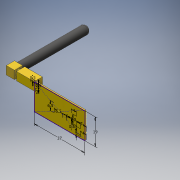
# Autodesk Inventor part: APC 220
Saved by Autodesk Inventor 2016 (Build 200138000, 138)
## iProperties
Created: 2016-05-08
Part Number: APC 220
Material: Generic
Document SubType Name: Modeling
Designer: Kenneth Daniel
Density: 1 g/cm^3
Appearance: Default
Author: Kenneth Daniel
Autodesk Inventor part; units mm, degrees
ref_plane "YZ Plane" through (0, 0, 0) normal (1, 0, 0) x (0, 1, 0)
ref_plane "XZ Plane" through (0, 0, 0) normal (0, 1, 0) x (-1, 0, 0)
ref_plane "XY Plane" through (0, 0, 0) normal (0, 0, 1) x (1, 0, 0)
sketch "Sketch1" plane through (0, 0, 0) normal (0, 1, 0) x (-1, 0, 0)
  line L0 (-18.5, 9.5) -> (-18.5, -9.5)
  line L1 (-18.5, -9.5) -> (18.5, -9.5)
  line L2 (18.5, -9.5) -> (18.5, 9.5)
  line L3 (18.5, 9.5) -> (-18.5, 9.5)
  line L4 (-18.5, 9.5) -> (18.5, -9.5) construction
  line L5 (-18.5, -9.5) -> (18.5, 9.5) construction
  point P0 (0, 0)
  dimension "d0" = 19
  dimension "d1" = 37
  constraints: 12 end point, 2 midpoint, 2 parallel, 1 perpendicular, 1 vertical
  measures "d0" distance of L0.start L0.end
  measures "d1" distance of L1.end L0.end
extrude "Extrusion1" add sketch "Sketch1" along normal blind 1
sketch "Sketch2" plane through (0, 1, 0) normal (0, 1, 0) x (1, 0, 0)
  line L0 (-18.5, 9.5) -> (-18.5, -9.5) construction
  line L1 (18.5, 9.5) -> (-18.5, 9.5) construction
  line L2 (-18.5, -9.5) -> (18.5, 9.5) construction
  line L3 (18.5, -9.5) -> (18.5, 9.5) construction
  line L4 (-18.5, 9.5) -> (18.5, -9.5) construction
  line L5 (-18.5, 0) -> (18.5, 0) construction
  line L6 (0, -9.5) -> (0, 9.5) construction
  line L7 (18.5, 9.5) -> (14.5, 9.5) construction
  line L8 (14.5, 9.5) -> (14.5, 8.5) construction
  line L9 (14.5, 8.5) -> (14.5, 4.5)
  line L10 (14.5, 4.5) -> (4.5, 4.5)
  line L11 (4.5, 4.5) -> (4.5, 8.5)
  line L12 (4.5, 8.5) -> (14.5, 8.5)
  line L13 (4.5, 4.5) -> (14.5, 8.5) construction
  line L14 (4.5, 8.5) -> (14.5, 4.5) construction
  line L15 (6.6893, 4.5) -> (6.6893, 8.5) construction
  line L16 (6.6893, 5.3757) -> (14.5, 5.3757) construction
  line L17 (12.159, 4.5) -> (12.159, 8.5) construction
  line L18 (6.6893, 6.5) -> (12.159, 6.5) construction
  line L19 (6.6893, 8.5) -> (12.159, 8.5)
  line L20 (12.159, 4.5) -> (6.6893, 4.5)
  arc A0 (6.6893, 8.5) -> (6.6893, 4.5) centre (6.6893, 6.5) ccw
  arc A1 (12.159, 4.5) -> (12.159, 8.5) centre (12.159, 6.5) ccw
  line L21 (18.5, 4.5) -> (11.5, 4.5) construction
  line L22 (11.5, 4.5) -> (11.5, 4) construction
  line L23 (11.5, 4) -> (11.5, -2)
  line L24 (11.5, -2) -> (7.5, -2)
  line L25 (7.5, -2) -> (7.5, 4)
  line L26 (7.5, 4) -> (11.5, 4)
  line L27 (7.5, 4) -> (1.5, 4) construction
  line L28 (1.5, 4) -> (-5, 4)
  line L29 (-5, 4) -> (-5, -2.5)
  line L30 (-5, -2.5) -> (1.5, -2.5)
  line L31 (1.5, -2.5) -> (1.5, 4)
  line L32 (-18.5, -9.5) -> (-18.5, -9)
  line L33 (-18.5, -9) -> (-18.5, -8)
  line L34 (-18.5, -8) -> (-18.5, -7.5)
  line L35 (-18.5, -7.5) -> (-18.5, -6.5)
  line L36 (-18.5, -6.5) -> (-18.5, -6)
  line L37 (-18.5, -6) -> (-18.5, -5)
  line L38 (-18.5, -5) -> (-16.5, -5)
  line L39 (-16.5, -5) -> (-16.5, -9)
  line L40 (-16.5, -9) -> (-18.5, -9)
  line L41 (-18.5, -8) -> (-16.5, -8)
  line L42 (-18.5, -7.5) -> (-16.5, -7.5)
  line L43 (-18.5, -6.5) -> (-16.5, -6.5)
  line L44 (-18.5, -6) -> (-16.5, -6)
  point P0 (0, 0)
  point P1 (9.4242, 6.5)
  dimension "d4" = 4
  dimension "d5" = 1
  dimension "d6" = 4
  dimension "d7" = 10
  dimension "d8" = 7
  dimension "d9" = 0.5
  dimension "d10" = 6
  dimension "d11" = 4
  dimension "d12" = 6
  dimension "d13" = 6.5
  dimension "d14" = 6.5
  dimension "d15" = 0.5
  dimension "d16" = 1
  dimension "d17" = 0.5
  dimension "d18" = 1
  dimension "d19" = 0.5
  dimension "d20" = 1
  dimension "d21" = 2
  constraints: 86 end point, 15 perpendicular, 14 point on line, 9 parallel, 5 midpoint, 4 point on circle, 4 tangent, 2 centre point, 2 vertical, 8 other
  measures "d4" distance of L1.start L7.end
  measures "d5" distance of L7.end L8.end
  measures "d6" distance of L8.end L9.end
  measures "d7" distance of L9.end L10.end
  measures "d8" distance of L21.start L21.end
  measures "d9" distance of L21.end L22.end
  measures "d10" distance of L22.end L23.end
  measures "d11" distance of L23.end L24.end
  measures "d12" distance of L25.end L27.end
  measures "d13" distance of L27.end L28.end
  measures "d14" distance of L29.end L28.end
  measures "d15" distance of L2.start L32.end
  measures "d16" distance of L32.end L33.end
  measures "d17" distance of L33.end L34.end
  measures "d18" distance of L34.end L35.end
  measures "d19" distance of L35.end L36.end
  measures "d20" distance of L36.end L37.end
  measures "d21" distance of L37.end L38.end
extrude "Extrusion2" add sketch "Sketch2" along normal blind 0.25 contours L9 L10 A1 L12 | A1 L10 A0 L12 | A0 L10 L11 L12 | L23 L24 L25 L26 | L31 L30 L29 L28
extrude "Extrusion3" add sketch "Sketch2" along normal blind 1 contours L33 L41 L39 L40 | L35 L43 L39 L42 | L37 L38 L39 L44
sketch "Sketch3" plane through (-18.5, 0, -9.5) normal (-1, 0, 0) x (0, 0, 1)
  line L0 (19, 0) -> (19, 1) projected
  line L1 (19, 0) -> (19, 6)
  line L2 (19, 6) -> (13, 6)
  line L3 (13, 6) -> (13, 0)
  line L4 (0, 0) -> (19, 0) projected
  point P0 (9.5, 0)
  dimension "d26" = 6
  dimension "d27" = 6
  constraints: 6 end point, 2 perpendicular, 1 collinear, 1 point on line
  measures "d26" distance of L0.start L1.end
  measures "d27" distance of L1.end L2.end
extrude "Extrusion4" add sketch "Sketch3" along normal blind 13
sketch "Sketch4" plane through (-31.5, 0, -9.5) normal (-1, 0, 0) x (0, 0, 1)
  line L0 (13, 6) -> (13, 1) construction
  line L1 (19, 0) -> (19, 1) construction
  line L2 (13, 6) -> (19, 0) construction
  line L3 (19, 0) -> (19, 6) construction
  line L4 (19, 6) -> (13, 0) construction
  circle A0 centre (16, 3) radius 2.25
  point P0 (9.5, 0)
  dimension "d30" = 4.5
  constraints: 6 end point, 1 centre point, 1 collinear, 1 midpoint, 1 perpendicular
  measures "d30" diameter of A0
extrude "Extrusion5" add sketch "Sketch4" along normal blind 1.5
sketch "Sketch5" plane through (-33, 3, 6.5) normal (-1, 0, 0) x (0, 0, 1)
  line L0 (3, -3) -> (3, 3)
  line L1 (3, 3) -> (-3, 3)
  line L2 (-3, 3) -> (-3, -3)
  line L3 (-3, -3) -> (3, -3)
  line L4 (3, -3) -> (-3, 3) construction
  line L5 (3, 3) -> (-3, -3) construction
  point P0 (-6.5, -3)
  point P1 (0, 0)
  dimension "d33" = 6
  dimension "d34" = 6
  constraints: 12 end point, 2 midpoint, 2 parallel, 1 perpendicular, 1 vertical
  measures "d33" distance of L0.start L0.end
  measures "d34" distance of L1.end L0.end
extrude "Extrusion6" add sketch "Sketch5" along normal blind 6
sketch "Sketch6" plane through (-33, 6, 9.5) normal (0, 1, 0) x (1, 0, 0)
  line L0 (-6, 0) -> (-6, 6) construction
  line L1 (-6, 6) -> (0, 0) construction
  line L2 (0, 0) -> (0, 6) construction
  line L3 (0, 6) -> (-6, 0) construction
  circle A0 centre (-3, 3) radius 3
  point P0 (33, 9.5)
  constraints: 6 end point, 1 centre point, 1 midpoint, 1 parallel, 1 perpendicular
extrude "Extrusion7" add sketch "Sketch6" along normal blind 50
fillet "Fillet1" radius 2 1 edges at (-39, 56, 6.5)
extrude "Extrusion8" add sketch "Sketch2" along normal blind 5 contours A1 L10 A0 L12
fillet "Fillet2" radius 0.5 4 edges at (9.4242, 6, -4.5) (14.159, 6, -6.5) (9.4242, 6, -8.5) (4.6893, 6, -6.5)
body "Solid1"
